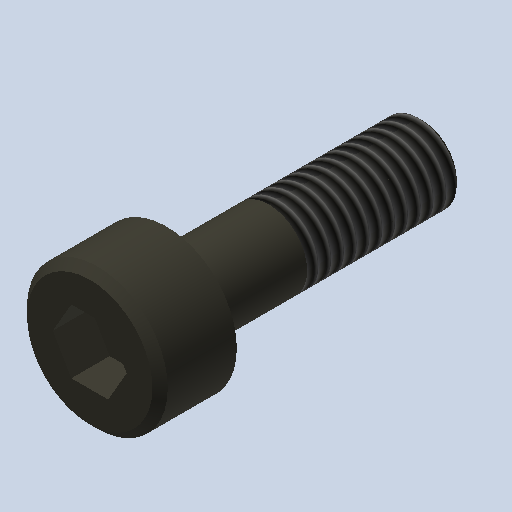
# Autodesk Inventor part: SCREW,SOCKET-HD,P,12_9,M03X0_5X10MM
Saved by Autodesk Inventor 2024.3 (Build 283343000, 343)
## iProperties
Category: _
Manager: 613-12338
Created: 2018-08-02
Part Number: SCREW,SOCKET-HD,P,12_9,M03X0_5X10MM
Checked By: 0002449373
Engr Approved By: P
User Status: Released
Material: Steel, MS
Description: SCREW,SOCKET-HD,P,12.9,M03X0.50X006MM
Document SubType Name: Modeling
Mfg Approved By: Cathy.Lesperance
Designer: Clint.Matte
Manufacturer: Standard
Standards Organization: Custom
Density: 7.86 g/cm^3
Appearance: Gunmetal
Mass: 0.823065 g
Surface Area: 1.64881 cm^2
Volume: 0.104716 cm^3
CN_MASS: 0.0
CN_SERVICEABLE: _
FIRST_DESCRIPTION: SOCKET HEAD CAP SCREW, STEEL 12.9
SECOND_DESCRIPTION: M3 x 0.5 x 6 MM
THIRD_DESCRIPTION: WV
PTC_WM_ITERATION: 6
PTC_WM_ORGANIZATION_ID: CLWC
PTC_WM_LIFECYCLE: CLWC_CAD_LC
CL_runCount: 1
ModelCat: Uncategorized
Subject: FMPSHMA030050006
Author: -
Keywords: GENERIC
Revision Number: A
Autodesk Inventor part; units mm, degrees
ref_plane "YZ Plane" through (0, 0, 0) normal (1, 0, 0) x (0, 1, 0)
ref_plane "XZ Plane" through (0, 0, 0) normal (0, 1, 0) x (-1, 0, 0)
ref_plane "XY Plane" through (0, 0, 0) normal (0, 0, 1) x (1, 0, 0)
sketch "Sketch3" plane through (0, 0, 0) normal (0, 0, 1) x (1, 0, 0)
  circle A0 centre (0, 0) radius 1.5
  dimension "Diameter" = 3
  constraints: 1 centre point, 1 coincident
  measures "Diameter" diameter of A0
extrude "Extrusion1" add sketch "Sketch3" against normal blind 10
sketch "Sketch4" plane through (0, 0, 0) normal (0, 0, 1) x (1, 0, 0)
  circle A0 centre (0, 0) radius 1.5 projected
  circle A1 centre (0, 0) radius 2.75
  dimension "Head_Diameter" = 5.5
  constraints: 1 centre point, 1 coincident
  measures "Head_Diameter" diameter of A1
extrude "Extrusion2" add sketch "Sketch4" along normal blind 3 contours A0 | A1
sketch "Sketch5" plane through (0, 0, 3) normal (0, 0, 1) x (1, 0, 0)
  circle A0 centre (0, 0) radius 2.75 projected
  line L0 (1.4434, 0) -> (0.7217, -1.25)
  line L1 (0.7217, -1.25) -> (-0.7217, -1.25)
  line L2 (-0.7217, -1.25) -> (-1.4434, 0)
  line L3 (-1.4434, 0) -> (-0.7217, 1.25)
  line L4 (-0.7217, 1.25) -> (0.7217, 1.25)
  line L5 (0.7217, 1.25) -> (1.4434, 0)
  line L6 (0, 0) -> (1.4434, 0) construction
  dimension "Hex_Width" = 2.5
  constraints: 14 end point, 1 coincident, 1 horizontal, 13 other
  measures "Hex_Width" distance between parallel lines of L1 L4
extrude "Extrusion3" cut sketch "Sketch5" against normal blind 1.5 contours L0 L1 L2 L3 L4 L5
thread "Thread1" size "M3x0.5" class "4g6g" standard "ANSI Metric M Profile" length 6
chamfer "Chamfer1" distance 0.3 angle 45 1 edges at (-2.75, 0, 3)
chamfer "Chamfer2" distance 0.15 angle 45 1 edges at (-1.5, 0, -10)
equation "\"d14\" = 0.5 * Chamfer"
equation "\"Chamfer\" = 0.3"
body "Solid1"
